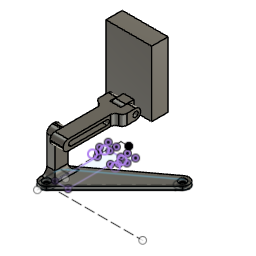
Fan Mount v1 (Autodesk Fusion 360 design; units mm, degrees)
Autodesk Fusion 360 part; units mm, degrees
sketch "Sketch1" plane through (0, 0, 0) normal (0, 1, 0) x (1, 0, 0)
  line L0 (0, 0) -> (14, 0) construction
  line L1 (14, 0) -> (-14, 0)
  line L2 (-14, 0) -> (-14, -40)
  line L3 (-14, -40) -> (14, -40)
  line L4 (14, -40) -> (14, 0)
  line L5 (0, 0) -> (3.175, 0)
  line L6 (3.175, 0) -> (-3.175, 0)
  line L7 (-3.175, 0) -> (-3.175, -6.35)
  line L8 (-3.175, -6.35) -> (3.175, -6.35)
  line L9 (3.175, -6.35) -> (3.175, 0)
  dimension "d1" = 14
  dimension "d2" = 28
  dimension "d3" = 40
  dimension "d4" = 3.175
  dimension "d5" = 6.35
  dimension "d6" = 6.35
  constraint coincident L0.start L5.start
  constraint horizontal L0
  constraint horizontal L1
  constraint vertical L2
  constraint horizontal L3
  constraint vertical L4
  constraint parallel L1 L5
  constraint horizontal L6
  constraint vertical L7
  constraint horizontal L8
  constraint vertical L9
  measures "d1" distance of L0.start L0.end
  measures "d2" distance of L0.end L1.end
  measures "d3" distance of L0.end L3.end
  measures "d4" distance of L0.start L5.end
  measures "d5" distance of L5.end L6.end
  measures "d6" distance of L5.end L8.end
extrude "Extrude2" add sketch "Sketch1" against normal blind 8 contours L1 L5 L6 L7 L8 L9 makes body 1
extrude "Extrude1" add sketch "Sketch1" along normal blind 10 separate body makes body 2
fillet "Fillet1" radius 3 2 edges at (0, -8, 6.35) (0, -8, 0) on bodies 1
hole "Hole1" at (-3.175, -5.003, 3.1862) direction (1, 0, 0) diameter 3 depth 9 tip angle 118 bodies 1
sketch "Sketch1 (2)" plane through (0, 0, 0) normal (0, 0, 1) x (1, 0, 0) in component "mount"
  line L0 (3.175, -5) -> (-3.175, -5)
  line L1 (-3.175, -5) -> (-3.175, 0)
  line L2 (-3.175, 0) -> (3.175, 0)
  line L3 (3.175, 0) -> (3.175, -5)
  line L4 (14, 0) -> (-14, 0)
  line L5 (-14, 0) -> (-14, 10)
  line L6 (-14, 10) -> (14, 10)
  line L7 (14, 10) -> (14, 0)
  line L8 (3.175, -5) -> (3.175, -8)
  line L9 (3.175, -8) -> (-3.175, -8)
  line L10 (-3.175, -8) -> (-3.175, -5)
  line L11 (-3.175, -5) -> (3.175, -5)
  line L12 (-3.375, -8.2) -> (-3.375, -5.2) construction
  line L13 (3.375, -4.8) -> (3.375, -8.2) construction
  line L14 (3.375, -8.2) -> (-3.375, -8.2) construction
  line L15 (-3.375, -5.2) -> (-3.375, 0.2) construction
  line L16 (-3.375, 0.2) -> (3.375, 0.2) construction
  line L17 (3.375, 0.2) -> (3.375, -5.2) construction
  line L18 (-3.375, -8.2) -> (3.375, -8.2)
  line L19 (3.375, -8.2) -> (3.375, -1.2)
  line L20 (3.375, -1.2) -> (-3.375, -1.2)
  line L21 (-3.375, -1.2) -> (-3.375, -8.2)
  line L22 (-3.375, -1.2) -> (-8.375, -1.2)
  line L23 (-8.375, -1.2) -> (-8.375, -12.4721)
  line L24 (3.375, -1.2) -> (8.375, -1.2)
  line L25 (8.375, -1.2) -> (8.375, -12.4721)
  line L26 (-8.375, -12.4721) -> (8.375, -12.4721)
  dimension "d18" = 7
  dimension "d19" = 5
  dimension "d20" = 5
  constraint parallel L10 L12
  constraint parallel L8 L13
  constraint parallel L9 L14
  constraint parallel L1 L15
  constraint parallel L2 L16
  constraint parallel L3 L17
  constraint horizontal L18
  constraint vertical L19
  constraint horizontal L20
  constraint vertical L21
  constraint coincident L17 L19.end
  constraint perpendicular L21 L22
  constraint perpendicular L18 L23
  constraint perpendicular L17 L24
  constraint perpendicular L24 L25
  constraint perpendicular L25 L26
  measures "d18" distance of L12.start L20.end
  measures "d19" distance of L20.end L22.end
  measures "d20" distance of L19.end L24.end
extrude "Extrude1'" add sketch "Sketch1 (2)" along normal blind 6.35 separate body contours L18 L19 L21 L22 L23 L24 L25 L26 makes body 3 in component "mount"
fillet "Fillet1'" radius 3 4 edges at (-5.875, -1.2, 6.35) (-5.875, -1.2, 0) (5.875, -1.2, 0) (5.875, -1.2, 6.35) on bodies 3 in component "mount"
ref_plane "WorkPlane1" through (0, -6.836, 3.175) normal (-1, 0, 0) x (0, -1, 0) in component "mount"
sketch "Sketch2" plane through (0, -6.836, 3.175) normal (-1, 0, 0) x (0, 1, 0) in component "mount"
  arc A0 (5.636, 0.175) -> (2.636, 3.175) centre (2.636, 0.175) ccw
  line L0 (2.636, 3.175) -> (-5.636, 3.175)
  line L1 (-5.636, 3.175) -> (-5.636, -3.175)
  line L2 (-5.636, -3.175) -> (2.636, -3.175)
  arc A1 (2.636, -3.175) -> (5.636, -0.175) centre (2.636, -0.175) ccw
  line L3 (5.636, -0.175) -> (5.636, 0.175)
  line L4 (2.636, -0.175) -> (2.636, 0.175)
  circle A2 centre (2.636, 0) radius 1.6
  line L5 (2.636, 0) -> (-29.364, 0) construction
  line L6 (-29.364, 0) -> (-29.364, 20) construction
  line L7 (-5.636, -3.175) -> (-34.364, -3.175)
  line L8 (-37.364, -0.175) -> (-37.364, 0.175)
  line L9 (-34.364, 3.175) -> (-5.636, 3.175)
  line L10 (-5.636, 3.175) -> (-5.636, -3.175) construction
  line L11 (-10.5, 1.5) -> (-32.5, 1.5)
  line L12 (-32.5, -1.5) -> (-10.5, -1.5)
  arc A3 (-37.364, -0.175) -> (-34.364, -3.175) centre (-34.364, -0.175) ccw
  arc A4 (-34.364, 3.175) -> (-37.364, 0.175) centre (-34.364, 0.175) ccw
  arc A5 (-32.5, 1.5) -> (-32.5, -1.5) centre (-32.5, 0) ccw
  arc A6 (-10.5, -1.5) -> (-10.5, 1.5) centre (-10.5, 0) ccw
  point P0 (-37.364, -3.175)
  point P1 (-21.5, 0)
  dimension "d25" = 3.2
  dimension "d26" = 32
  dimension "d27" = 20
  dimension "d28" = 31.728
  dimension "d29" = 22
  dimension "d30" = 3
  dimension "d31" = 3
  dimension "d32" = 3
  constraint coincident A1.centre L4.start
  constraint coincident A0.centre L4.end
  constraint midpoint L4 A2.centre
  constraint coincident A2.centre L5.start
  constraint perpendicular L4 L5
  constraint perpendicular L5 L6
  constraint horizontal L7
  constraint vertical L8
  constraint horizontal L9
  constraint vertical L10
  constraint coincident L1.end L2.start
  constraint coincident L0.end L9
  constraint horizontal L11
  constraint parallel L11 L12
  constraint coincident P0 L7
  constraint coincident P0 L8
  constraint tangent L7 A3
  constraint tangent L8 A3
  constraint tangent L9 A4
  constraint tangent L8 A4
  measures "d25" diameter of A2
  measures "d26" distance of A2.centre L5.end
  measures "d27" distance of L5.end L6.end
  measures "d28" distance of L1.end P0
  measures "d29" distance of L12.start L12.end
  measures "d30" distance of L11.end L12.start
  measures "d31" radius of A3
  measures "d32" radius of A4
extrude "Extrude3" cut sketch "Sketch2" along normal mid plane 16.75 contours A2 bodies 3 in component "mount"
extrude "Extrude2'" add sketch "Sketch2" along normal mid plane 8 contours L1 L7 L8 L9 A3 A4 bodies 3 in component "mount"
fillet "Fillet2" radius 3 2 edges at (-8.375, -12.4721, 3.175) (8.375, -12.4721, 3.175) on bodies 3 in component "mount"
fillet "Fillet3" radius 3 2 edges at (-4, -12.4721, 3.175) (4, -12.4721, 3.175) on bodies 3 in component "mount"
ref_plane "WorkPlane2" through (0, 0, -20) normal (0, 0, 1) x (1, 0, 0) in component "mount"
sketch "Sketch3" plane through (0, 0, -20) normal (0, 0, 1) x (1, 0, 0) in component "mount"
  line L0 (4, -15.2478) -> (4, -41.2001)
  line L1 (4, -41.2001) -> (-4, -41.2001)
  line L2 (-4, -41.2001) -> (-4, -15.2478)
  arc A0 (-4, -15.2478) -> (-6.1875, -12.36) centre (-7, -15.2478) ccw
  arc A1 (-8.375, -9.4721) -> (-6.1875, -12.36) centre (-5.375, -9.4721) ccw
  line L3 (-8.375, -9.4721) -> (-8.375, -4.2)
  line L4 (-8.375, -4.2) -> (-3.375, -4.2)
  line L5 (-3.375, -4.2) -> (-3.375, -8.2)
  line L6 (-3.375, -8.2) -> (3.375, -8.2)
  line L7 (3.375, -8.2) -> (3.375, -4.2)
  line L8 (3.375, -4.2) -> (8.375, -4.2)
  line L9 (8.375, -4.2) -> (8.375, -9.4721)
  arc A2 (6.1875, -12.36) -> (8.375, -9.4721) centre (5.375, -9.4721) ccw
  arc A3 (6.1875, -12.36) -> (4, -15.2478) centre (7, -15.2478) ccw
  line L10 (0, 0) -> (-4.8, 0) construction
  line L11 (-4, -41.2001) -> (-9, -41.2001)
  line L12 (-9, -41.2001) -> (-9, -36.7143)
  line L13 (-8.054, -33.2001) -> (-4, -33.2001)
  line L14 (-4, -33.2001) -> (-4, -41.2001)
  line L15 (-4.8, 0) -> (-4.8, -51.1867) construction
  line L16 (-4.8, -41.2001) -> (-4.8, -45.7001) construction
  circle A4 centre (-4.8, -45.7001) radius 2.25
  line L17 (-4.8, -45.7001) -> (36.9193, -3.9808) construction
  line L18 (-4.8, -45.7001) -> (54.2, -45.7001) construction
  circle A5 centre (36.9193, -3.9808) radius 2.25
  circle A6 centre (-4.8, -45.7001) radius 4
  circle A7 centre (36.9193, -3.9808) radius 4
  line L19 (-9, -41.2001) -> (-8.7962, -45.8743)
  line L20 (4.1782, -42.3787) -> (37.5412, -9.0157)
  line L21 (4.1782, -42.3787) -> (-1.9716, -48.5285)
  line L22 (37.5412, -9.0157) -> (39.7477, -6.8092)
  line L23 (-6.1818, -31.1007) -> (34.5297, -0.773)
  arc A8 (-6.1818, -31.1007) -> (-9, -36.7143) centre (-2, -36.7143) ccw
  dimension "d42" = 4.8
  dimension "d43" = 5
  dimension "d44" = 8
  dimension "d45" = 4.5
  dimension "d46" = 4.5
  dimension "d47" = 45
  dimension "d48" = 59
  dimension "d49" = 4.5
  dimension "d50" = 8
  dimension "d51" = 8
  dimension "d52" = 7
  constraint coincident L10.start origin
  constraint perpendicular L5 L10
  constraint horizontal L11
  constraint vertical L12
  constraint horizontal L13
  constraint vertical L14
  constraint coincident L1.end L2.start
  constraint perpendicular L6 L15
  constraint coincident L11 L16.start
  constraint coincident L15 L16.start
  constraint perpendicular L11 L16
  constraint coincident L16.end A4.centre
  constraint horizontal L18
  constraint coincident L17.end A5.centre
  constraint concentric A4 A6
  constraint concentric A5 A7
  constraint coincident A6 L19.end
  constraint tangent A6 L19
  constraint tangent A6 L20
  constraint tangent A7 L20
  constraint coincident A6 L21.end
  constraint tangent A6 L21
  constraint parallel L20 L21
  constraint coincident A7 L22.end
  constraint tangent A7 L22
  constraint parallel L20 L22
  constraint coincident A7 L23.end
  constraint tangent A7 L23
  constraint tangent L12 A8
  constraint tangent L23 A8
  constraint coincident A8 L13.start
  measures "d42" distance of L10.start L10.end
  measures "d43" distance of L1.end L11.end
  measures "d44" distance of L1.end L13.end
  measures "d45" distance of L16.start L16.end
  measures "d46" diameter of A4
  measures "d47" angle of L17 L18
  measures "d48" distance of L16.end L17.end
  measures "d49" diameter of A5
  measures "d50" diameter of A6
  measures "d51" diameter of A7
  measures "d52" radius of A8
extrude "Extrude5" add sketch "Sketch3" along normal blind 26.35 separate body contours L2 L11 L12 L13 L14 A8 makes body 4 in component "mount"
extrude "Extrude4" add sketch "Sketch3" along normal blind 2 separate body contours L0 L1 L11 A6 A7 L19 L20 L21 L22 L23 | L0 L1 L2 L14 L23 | L2 L13 L23 A8 | A7 | L2 L11 L12 L13 L14 A8 | A6 makes body 5 in component "mount"
fillet "Fillet4" radius 3.5 2 edges at (-6.027, -33.2001, 6.35) (-6.5, -41.2001, 6.35) on bodies 4 in component "mount"
combine "Combine1" operation add target body 4 tool bodies 5 in component "mount"
fillet "Fillet5" radius 3.5 3 edges at (-6.5, -41.2001, -18) (-4, -37.2001, -18) (-6.027, -33.2001, -18) on bodies 4 in component "mount"
sketch "Sketch4" plane through (-9, 0, 0) normal (-1, 0, 0) x (0, -1, 0) in component "mount"
  line L0 (41.2001, -20) -> (41.2001, -14.5)
  line L1 (41.2001, -14.5) -> (41.2001, 2.85)
  arc A0 (41.2001, 2.85) -> (37.7001, 6.35) centre (37.7001, 2.85) ccw
  line L2 (37.7001, 6.35) -> (36.7143, 6.35)
  line L3 (36.7143, 6.35) -> (36.7143, -20)
  line L4 (36.7143, -20) -> (41.2001, -20)
  line L5 (15.2478, 6.35) -> (15.2478, 0)
  line L6 (15.2478, 0) -> (41.2001, 0)
  arc A1 (41.2001, 0) -> (44.2001, 3) centre (41.2001, 3) ccw
  line L7 (44.2001, 3) -> (44.2001, 3.35)
  arc A2 (44.2001, 3.35) -> (41.2001, 6.35) centre (41.2001, 3.35) ccw
  line L8 (41.2001, 6.35) -> (15.2478, 6.35)
  arc A3 (17.3361, 4.675) -> (17.3361, 1.675) centre (17.3361, 3.175) ccw
  line L9 (17.3361, 4.675) -> (39.3361, 4.675)
  arc A4 (39.3361, 1.675) -> (39.3361, 4.675) centre (39.3361, 3.175) ccw
  line L10 (39.3361, 1.675) -> (17.3361, 1.675)
  line L11 (36.7143, -20) -> (36.7143, 6.35)
  line L12 (36.7143, 6.35) -> (36.7001, 6.35)
  spline S0 degree 3 poles (33.2001, 2.85) (33.2001, 3.2991) (33.2915, 3.771) (33.6507, 4.6299) (33.9183, 5.0179) (34.5309, 5.6306) (34.9192, 5.8989) (35.7795, 6.2588) (36.2521, 6.35) (36.7001, 6.35) knots 1.076295 1.076295 1.076295 1.076295 1.21103 1.21103 1.345764 1.345764 1.480176 1.480176 1.614587 1.614587 1.614587 1.614587
  line L13 (33.2001, 2.85) -> (33.2001, -14.5)
  spline S1 degree 3 poles (31.1007, -17.7075) (31.1674, -17.6784) (31.2351, -17.6464) (31.4729, -17.5238) (31.6657, -17.406) (32.0475, -17.1074) (32.2357, -16.9256) (32.6244, -16.4562) (32.838, -16.1048) (33.1262, -15.327) (33.2001, -14.901) (33.2001, -14.5) knots 2.182489 2.182489 2.182489 2.182489 2.216653 2.216653 2.300783 2.300783 2.384913 2.384913 2.505202 2.505202 2.625491 2.625491 2.625491 2.625491
  line L14 (31.1007, -17.7075) -> (31.1007, -20)
  line L15 (36.7143, -20) -> (31.1007, -20)
  line L16 (33.2001, 3.175) -> (41.2001, 3.175) construction
  line L17 (37.2001, 4.675) -> (37.2001, 1.675) construction
  circle A5 centre (37.2001, 3.175) radius 1.5
  constraint coincident L13 L16.start
  constraint coincident L1 L16.end
  constraint perpendicular L1 L16
  constraint coincident L9 L17.start
  constraint coincident L10 L17.end
  constraint perpendicular L10 L17
  constraint midpoint L16 L17
  constraint midpoint L16 A5.centre
  constraint coincident L17.end A5
extrude "Extrude6" cut sketch "Sketch4" against normal blind 5 contours L3 L11 A5 | L3 L11 A5 bodies 4 in component "mount"
component "mount" placed x (1, 0, 0) y (0, 1, 0) z (0, 0, 1) at (0, 0, 0)
equation "d28 = 40 mm - 8.272 mm"
